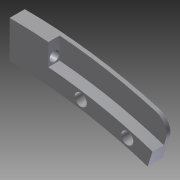
# Autodesk Inventor part: FiberClamper_v2
Saved by Autodesk Inventor 2012 SP2 (Build 160219200, 219)
## iProperties
Created: 2015-03-09
Part Number: FiberClamper_v2
Material: Default
Document SubType Name: Modeling
Designer: zhaox11
Density: 1 g/cm^3
Author: zhaox11
Autodesk Inventor part; units mm, degrees
ref_plane "YZ Plane" through (0, 0, 0) normal (1, 0, 0) x (0, 1, 0)
ref_plane "XZ Plane" through (0, 0, 0) normal (0, 1, 0) x (-1, 0, 0)
ref_plane "XY Plane" through (0, 0, 0) normal (0, 0, 1) x (1, 0, 0)
sketch "Sketch1" plane through (0, 0, 0) normal (0, 0, 1) x (1, 0, 0)
  line L0 (0, 0) -> (0, -93.6625)
  line L1 (0, 0) -> (0, 7.9375)
  arc A0 (31.3961, 2.9648) -> (0, 7.9375) centre (0, -93.6625) ccw
  arc A1 (28.9433, -4.5842) -> (0, 0) centre (0, -93.6625) ccw
  line L2 (0, -93.6625) -> (35.0444, 14.1931)
  line L3 (14.9183, 0.5277) -> (0, -93.6625)
  line L4 (14.9183, 0.5277) -> (26.5201, -1.3098)
  circle A2 centre (14.9183, 0.5277) radius 1.27
  line L5 (0, -93.6625) -> (24.6821, -1.5477)
  line L6 (24.6821, -1.5477) -> (28.1101, -2.4662)
  circle A3 centre (24.6821, -1.5477) radius 1.27
  dimension "d0" = 93.6625
  dimension "d1" = 7.9375
  dimension "d2" = 18
  dimension "d5" = 9
  dimension "d28" = 95.3643
  dimension "d29" = 2.54
  dimension "d32" = 6
  dimension "d33" = 95.3643
  dimension "d34" = 2.54
  constraints: 14 end point, 4 centre point, 4 coincident, 4 point on circle, 2 perpendicular, 2 point on line, 1 collinear, 1 vertical
  measures "d0" distance of L0.start L0.end
  measures "d1" distance of L0.start L1.end
  measures "d2" angle of L2 L0
  measures "d5" angle of L0 L3
  measures "d28" distance from line of L0.end L4
  measures "d29" diameter of A2
  measures "d32" angle of L5 L3
  measures "d33" distance from line of L0.end L6
  measures "d34" diameter of A3
extrude "Extrusion2" add sketch "Sketch1" along normal blind 3.175 contours L1 A0 L2 A1 L5 A3 L4 A2 L3 | L3 A2 L4 A3 L5 A1 | A2 L4 L3 | L3 L4 A2 | A3 L4 L6 L5 | L5 L6 A3 | A3 L4
sketch "Sketch3" plane through (0, 0, 0) normal (-1, 0, 0) x (0, 0, 1)
  line L0 (3.175, 0) -> (3.175, 7.9375) projected
  line L1 (0, 0) -> (3.175, 0) projected
  line L2 (0, 7.9375) -> (3.175, 7.9375)
  line L3 (3.175, 7.9375) -> (3.175, 3.048)
  line L4 (3.175, 3.048) -> (0, 3.048)
  line L5 (0, 3.048) -> (0, 7.9375)
  dimension "d13" = 3.048
  constraints: 8 end point, 2 parallel, 1 horizontal, 1 perpendicular, 1 point on line
  measures "d13" distance between parallel lines of L1 L4
extrude "Extrusion3" cut sketch "Sketch3" against normal blind 8.128
sketch "Sketch4" plane through (8.128, 0, 0) normal (-1, 0, 0) x (0, 0, 1)
  line L0 (0, 3.048) -> (0, 7.6119) projected
  line L1 (0, 3.048) -> (3.175, 3.048) projected
  line L2 (3.175, 7.6119) -> (3.175, 3.048) projected
  line L3 (3.175, 7.6119) -> (0.8128, 7.6119)
  line L4 (0.8128, 7.6119) -> (0.8128, 3.048)
  line L5 (0.8128, 3.048) -> (3.175, 3.048)
  line L6 (3.175, 3.048) -> (3.175, 7.6119)
  point P0 (0, 0)
  dimension "d16" = 0.8128
  constraints: 8 end point, 2 parallel, 1 horizontal, 1 perpendicular, 1 point on line
  measures "d16" distance between parallel lines of L4 L0
sketch3d "3D Sketch1"
  arc A0 (8.128, 7.6119, 0) -> (31.3961, 2.9648, 0) centre (0, -93.6625, 0) ccw
sweep "Sweep1" cut profiles "Sketch4" path "3D Sketch1"
sketch "Sketch5" plane through (0, 3.048, 3.175) normal (0, 1, 0) x (1, 0, 0)
  line L0 (0, 3.175) -> (8.128, 3.175)
  line L1 (8.128, 3.175) -> (8.128, 0)
  line L2 (8.128, 0) -> (0, 0)
  line L3 (0, 0) -> (0, 3.175)
  constraints: 8 end point, 2 parallel, 1 horizontal, 1 perpendicular
extrude "Extrusion4" add sketch "Sketch5" along normal blind 4.8895
sketch "Sketch6" plane through (0, 0, 0) normal (-1, 0, 0) x (0, 0, 1)
  line L0 (0, 7.9375) -> (3.175, 7.9375)
  line L1 (3.175, 7.9375) -> (3.175, 8.7188)
  line L2 (3.175, 8.7188) -> (0, 8.7188)
  line L3 (0, 8.7188) -> (0, 7.9375)
  constraints: 8 end point, 2 parallel, 1 horizontal, 1 perpendicular
sweep "Sweep2" cut profiles "Sketch6" path "Sketch1" path curves L1 A0
sketch "Sketch7" plane through (0, 0, 0) normal (-1, 0, 0) x (0, 0, 1)
  line L0 (0, 0) -> (3.175, 0) projected
  circle A0 centre (1.905, 4.3942) radius 1.016
  line L1 (3.175, 0) -> (3.175, 7.9375) projected
  dimension "d21" = 2.032
  dimension "d22" = 4.3942
  dimension "d25" = 1.27
  constraints: 1 centre point
  measures "d21" diameter of A0
  measures "d22" distance from line of L0 A0.centre
  measures "d25" distance from line of L1 A0.centre
extrude "Extrusion5" cut sketch "Sketch7" against normal blind 50.8
sketch "Sketch8" plane through (8.128, 3.048, 3.175) normal (1, 0, 0) x (0, 0, -1)
  circle A0 centre (1.27, 1.3462) radius 1.016 projected
  line L0 (2.3622, 4.5639) -> (0, 4.5639) projected
  line L1 (0, 0) -> (0, 4.5639) projected
  line L2 (2.3622, 0) -> (0, 0) projected
  line L3 (2.3622, 0) -> (2.3622, 4.5639) projected
  point P0 (3.175, -3.048)
  dimension "d26" = 1.3462
  measures "d26" distance from line of L2 A0.centre
fillet "Fillet1" radius 3.175 1 edges at (31.3961, 2.9648, 0.4064)
extrude "Extrusion9" cut sketch "Sketch1" along normal blind 12.7 contours A2 L4 L3 | L3 L4 A2 | A3 L4 L6 L5 | L5 L6 A3 | A3 L4
sketch "Sketch10" plane through (0, 0, 3.175) normal (0, 0, 1) x (1, 0, 0)
  circle A0 centre (24.6821, -1.5477) radius 1.27 projected
  circle A1 centre (14.9183, 0.5277) radius 1.27 projected
  arc A2 (8.128, 7.6119) -> (0, 7.9375) centre (0, -93.6625) ccw projected
  line L0 (0, 0) -> (0, 7.9375) projected
  arc A3 (28.9433, -4.5842) -> (0, 0) centre (0, -93.6625) ccw projected
  line L1 (29.9905, -1.3611) -> (28.9433, -4.5842) projected
  arc A4 (29.9905, -1.3611) -> (8.128, 3.048) centre (0, -93.6625) ccw projected
  line L2 (8.128, 3.048) -> (8.128, 7.6119) projected
  dimension "d45" = 14.9183
  dimension "d46" = 24.6821
  dimension "d47" = 0.5277
  dimension "d48" = 1.5477
  measures "d45" distance from line of L0 A1.centre
  measures "d46" distance from line of L0 A0.centre
  measures "d47" vertical distance of L0.start A1.centre
  measures "d48" vertical distance of L0.start A0.centre
equation "\"d33\" = d28"
body "Solid2"
